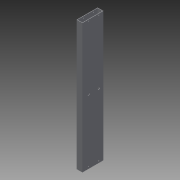
# Autodesk Inventor part: X Rail square
Saved by Autodesk Inventor 2013 SP2 (Build 170200200, 200)
## iProperties
Created: 2017-05-24
Part Number: X Rail square
Material: Generic
Document SubType Name: Modeling
Designer: Herman de Vries
Density: 1 g/cm^3
Author: Herman de Vries
Autodesk Inventor part; units mm, degrees
ref_plane "YZ Plane" through (0, 0, 0) normal (1, 0, 0) x (0, 1, 0)
ref_plane "XZ Plane" through (0, 0, 0) normal (0, 1, 0) x (-1, 0, 0)
ref_plane "XY Plane" through (0, 0, 0) normal (0, 0, 1) x (1, 0, 0)
sketch "Sketch1" plane through (0, 0, 0) normal (0, 0, 1) x (1, 0, 0)
  line L0 (0, 0) -> (18, 0)
  line L1 (18, 0) -> (18, 65)
  line L2 (18, 65) -> (0, 65)
  line L3 (0, 65) -> (0, 0)
  line L4 (1.5, 63.5) -> (16.5, 63.5)
  line L5 (16.5, 63.5) -> (16.5, 1.5)
  line L6 (16.5, 1.5) -> (1.5, 1.5)
  line L7 (1.5, 1.5) -> (1.5, 63.5)
  dimension "d0" = 18
  dimension "d1" = 65
  dimension "d2" = 1.5
  constraints: 16 end point, 4 parallel, 2 perpendicular, 1 horizontal, 3 other
  measures "d0" distance of L2.end L1.end
  measures "d1" distance of L1.end L0.end
  measures "d2" distance between parallel lines of L3 L7
extrude "Extrusion1" add sketch "Sketch1" along normal blind 400
sketch "Sketch2" plane through (0, 0, 0) normal (-1, 0, 0) x (0, 0, 1)
  line L0 (0, 65) -> (400, 65) projected
  circle A0 centre (6, 50.5) radius 1.65 projected
  circle A1 centre (6, 19.5) radius 1.5 projected
  circle A2 centre (396, 19.5) radius 1.65 projected
  circle A3 centre (396, 50.5) radius 1.65 projected
  circle A4 centre (200, 50.5) radius 4
  circle A5 centre (200, 19.5) radius 4
  point P0 (200, 65)
  dimension "d5" = 8
  dimension "d7" = 8
  constraints: 2 centre point, 2 horizontal alignment, 2 vertical alignment, 1 midpoint
  measures "d5" diameter of A4
  measures "d7" diameter of A5
extrude "Extrusion2" cut sketch "Sketch2" against normal blind 20
equation "\"d7\" = d5"
body "Solid1"
